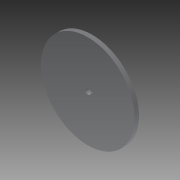
# Autodesk Inventor part: Platw_Wheel
Saved by Autodesk Inventor 2013 (Build 170138000, 138)
## iProperties
Created: 2015-07-07
Part Number: Platw_Wheel
Material: Polycarbonate, Clear
Document SubType Name: Modeling
Designer: Kyle
Density: 1.2 g/cm^3
Mass: 5.72253 g
Surface Area: 44.3831 cm^2
Volume: 4.76877 cm^3
Author: Kyle
Autodesk Inventor part; units mm, degrees
ref_plane "YZ Plane" through (0, 0, 0) normal (1, 0, 0) x (0, 1, 0)
ref_plane "XZ Plane" through (0, 0, 0) normal (0, 1, 0) x (-1, 0, 0)
ref_plane "XY Plane" through (0, 0, 0) normal (0, 0, 1) x (1, 0, 0)
sketch "Sketch1" plane through (0, 0, 0) normal (0, 0, 1) x (1, 0, 0)
  circle A0 centre (0, 0) radius 25.4
  circle A1 centre (0, 0) radius 1.6002
  dimension "d0" = 50.8
  dimension "d2" = 3.2004
  constraints: 2 centre point, 2 coincident
  measures "d0" diameter of A0
  measures "d2" diameter of A1
extrude "Extrusion1" add sketch "Sketch1" along normal blind 2.3622
body "Solid1"
